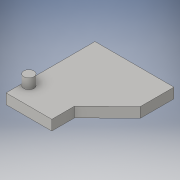
# Autodesk Inventor part: handmove
Saved by Autodesk Inventor 2016 (Build 200138000, 138)
## iProperties
Created: 2018-01-10
Part Number: handmove
Material: Generic
Document SubType Name: Modeling
Designer: New User
Density: 1 g/cm^3
Appearance: Default
Author: New User
Autodesk Inventor part; units mm, degrees
ref_plane "YZ Plane" through (0, 0, 0) normal (1, 0, 0) x (0, 1, 0)
ref_plane "XZ Plane" through (0, 0, 0) normal (0, 1, 0) x (-1, 0, 0)
ref_plane "XY Plane" through (0, 0, 0) normal (0, 0, 1) x (1, 0, 0)
sketch "Sketch1" plane through (0, 0, 0) normal (0, 1, 0) x (-1, 0, 0)
  line L0 (0, 0) -> (-197.3834, 0)
  line L1 (-197.3834, 0) -> (-197.3834, 84.1502)
  line L2 (-197.3834, 84.1502) -> (-114.3, 165.1)
  line L3 (-114.3, 165.1) -> (-114.3, 222.25)
  line L4 (-114.3, 222.25) -> (0, 222.25)
  line L5 (0, 222.25) -> (0, 0)
  dimension "d9" = 197.3834
  dimension "d10" = 222.25
  dimension "d11" = 84.1502
  dimension "d12" = 114.3
  dimension "d13" = 57.15
  constraints: 12 end point, 3 perpendicular, 1 horizontal, 1 parallel
  measures "d9" distance of L0.start L0.end
  measures "d10" distance of L4.end L0.start
  measures "d11" distance of L0.end L1.end
  measures "d12" distance of L3.end L4.end
  measures "d13" distance of L2.end L3.end
extrude "Extrusion1" add sketch "Sketch1" along normal blind 25.4
sketch "Sketch2" plane through (0, 25.4, 0) normal (0, 1, 0) x (1, 0, 0)
  circle A0 centre (12.7, -177.8) radius 12.7
  line L0 (0, -222.25) -> (114.3, -222.25) projected
  line L1 (0, 0) -> (0, -222.25) projected
  dimension "d14" = 44.45
  dimension "d15" = 25.4
  dimension "d16" = 12.7
  constraints: 1 centre point
  measures "d14" distance from line of L0 A0.centre
  measures "d15" diameter of A0
  measures "d16" distance from line of A0.centre L1
extrude "Extrusion2" add sketch "Sketch2" along normal blind 25.4
body "Solid1"
